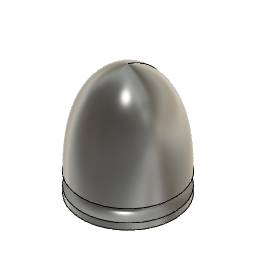
ShaanYadav_SpinningTop (Autodesk Fusion 360 design; units mm, degrees)
Autodesk Fusion 360 part; units mm, degrees
note: some values were not read from the file. Set by a fixed rule: which sketch regions a step uses.
sketch "Sketch1" plane through (0, 0, 0) normal (1, 0, 0) x (0, 1, 0)
  line L0 (0, 0) -> (0, 38.1)
  line L1 (0, 0) -> (0, -7.62)
  line L2 (0, 0) -> (19.05, 0)
  spline S0 degree 5 poles (0, 38.1) (0.8, 37.8209) (2.3616, 37.2184) (4.5883, 36.1814) (7.3226, 34.5283) (10.3245, 31.9824) (12.8801, 28.9222) (14.9644, 25.3189) (16.5831, 21.1789) (17.7714, 16.5429) (18.5698, 11.4576) (18.9259, 7.0635) (19.0446, 3.5971) (19.059, 1.2115) (19.05, 0) knots 0 0 0 0 0 0 0.1 0.2 0.3 0.4 0.5 0.6 0.7 0.8 0.9 1 1 1 1 1 1
  line L3 (0, -7.62) -> (2.54, -7.62)
  spline S1 degree 5 poles (2.54, -7.62) (2.6043, -7.4125) (2.746, -7.017) (2.9975, -6.4825) (3.4121, -5.8893) (4.0704, -5.3587) (4.8776, -5.0526) (5.8396, -4.9797) (6.9501, -5.1306) (8.1961, -5.4856) (9.5635, -6.0236) (10.7449, -6.5858) (11.6768, -7.0765) (12.3181, -7.4338) (12.6437, -7.62) knots 0 0 0 0 0 0 0.1 0.2 0.3 0.4 0.5 0.6 0.7 0.8 0.9 1 1 1 1 1 1
  line L4 (12.6437, -7.62) -> (18.9937, -7.62)
  line L5 (18.9937, -7.62) -> (18.9937, -5.08)
  spline S2 degree 5 poles (18.9937, -5.08) (18.7078, -4.978) (18.1611, -4.774) (17.4163, -4.4682) (16.5762, -4.0606) (15.7984, -3.5515) (15.3173, -3.0429) (15.1569, -2.5346) (15.33, -2.0269) (15.8233, -1.5195) (16.6124, -1.0126) (17.4609, -0.6074) (18.2117, -0.3036) (18.7622, -0.1012) (19.05, 0) knots 0 0 0 0 0 0 0.1 0.2 0.3 0.4 0.5 0.6 0.7 0.8 0.9 1 1 1 1 1 1
  point P0 (13.781, 27.1949)
  point P1 (5.08, -5.08)
  point P2 (15.24, -2.54)
  dimension "d1" = 7.62
  dimension "d2" = 19.05
  dimension "d5" = 6.35
  constraint coincident L0.start L1.start
  constraint vertical L0
  constraint parallel L0 L1
  constraint perpendicular L1 L2
  constraint perpendicular L1 L3
  constraint horizontal L4
  constraint perpendicular L4 L5
  measures "d1" distance of L0.start L1.end
  measures "d2" distance of L0.start L2.end
  measures "d5" distance of S1.end L4.end
revolve "Revolve1" add sketch "Sketch1" angle 360 about axis through (0, 0, 0) along (0, 0, 1)
